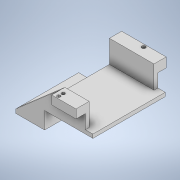
# Autodesk Inventor part: tray2
Saved by Autodesk Inventor 2020 (Build 240168000, 168)
## iProperties
Created: 2022-07-19
Part Number: tray2
Material: 일반
Document SubType Name: Modeling
Designer: SeungJin
Density: 1 g/cm^3
Appearance: 기본값
Author: SeungJin
Autodesk Inventor part; units mm, degrees
ref_plane "YZ Plane" through (0, 0, 0) normal (1, 0, 0) x (0, 1, 0)
ref_plane "XZ Plane" through (0, 0, 0) normal (0, 1, 0) x (-1, 0, 0)
ref_plane "XY Plane" through (0, 0, 0) normal (0, 0, 1) x (1, 0, 0)
sketch "스케치1" plane through (0, 0, 0) normal (0, 1, 0) x (-1, 0, 0)
  line L0 (70.5, 0) -> (70.5, 50)
  line L1 (70.5, 50) -> (0, 50)
  line L2 (0, 50) -> (0, 0)
  line L3 (24.5, 232.5) -> (-40, 232.5)
  line L4 (10, 242.5) -> (37.5, 242.5)
  line L5 (10, 232.5) -> (10, 242.5)
  line L6 (145.5, 232.5) -> (85.5, 232.5)
  line L7 (145.5, 242.5) -> (145.5, 232.5)
  line L8 (85.5, 242.5) -> (145.5, 242.5)
  line L9 (85.5, 232.5) -> (85.5, 242.5)
  line L10 (145.5, 0) -> (145.5, 242.5)
  line L11 (145.5, 242.5) -> (0, 242.5)
  line L12 (0, 242.5) -> (0, 0)
  line L13 (0, 50) -> (145.5, 50)
  circle A0 centre (93.5, 13) radius 2.067
  circle A1 centre (93.5, 37) radius 2.067
  circle A2 centre (147.5, 37) radius 2.067
  circle A3 centre (147.5, 13) radius 2.067
  line L14 (70.5, 0) -> (70.5, 50)
  line L15 (145.5, 50) -> (145.5, 81)
  line L16 (145.5, 75) -> (70.5, 75)
  line L17 (70.5, 50) -> (70.5, 75)
  line L18 (0, 0) -> (0, 25)
  line L19 (145.5, 27.5) -> (0, 27.5)
  line L20 (145.5, 0) -> (145.5, 25)
  line L21 (60.5, 242.5) -> (60.5, 267.5)
  line L22 (60.5, 267.5) -> (27.5, 267.5)
  line L23 (27.5, 267.5) -> (-42.5, 267.5)
  line L24 (145.5, 65) -> (-40, 65)
  circle A4 centre (12.5, 35) radius 2.067
  circle A5 centre (12.5, 15) radius 2.067
  circle A6 centre (-25, 256.5) radius 4.188
  circle A7 centre (12.5, 261) radius 2.067
  circle A8 centre (12.5, 249) radius 2.067
  line L25 (27.5, 242.5) -> (60.5, 242.5)
  line L26 (-40, 242.5) -> (20.5, 242.5)
  line L27 (0, 27.5) -> (0, 65)
  line L28 (145.5, 65) -> (145.5, 27.5)
  line L29 (0, 0) -> (145.5, 0)
  line L30 (24.5, 242.5) -> (24.5, 232.5)
  line L31 (0.5, 232.5) -> (0.5, 242.5)
  line L32 (113.5, 285) -> (113.5, 189)
  line L33 (39.5, 232.5) -> (39.5, 242.5)
  line L34 (39.5, 232.5) -> (24.5, 232.5)
  line L35 (-40, 242.5) -> (-40, 65)
  line L36 (-17.5, 242.5) -> (-17.5, 232.5)
  line L37 (0, 50) -> (-40, 50)
  line L38 (-40, 50) -> (-40, 65)
  line L39 (78.5, 75) -> (78.5, 0)
  point P0 (0, 227.5)
  point P1 (70.5, -15)
  point P2 (145.5, 227.5)
  point P3 (85.5, 242.5)
  point P4 (27.5, 242.5)
  point P5 (70.5, 25)
  point P6 (-5, 242.5)
  point P7 (0, 50)
  point P8 (70.5, 65)
  point P9 (0, 50)
  point P10 (78.5, 50)
  dimension "d1" = 50
  dimension "d3" = 4.134
  dimension "d4" = 4.134
  dimension "d5" = 4.134
  dimension "d6" = 4.134
  dimension "d7" = 12
  dimension "d8" = 12
  dimension "d9" = 32
  dimension "d10" = 15
  dimension "d29" = 40
  dimension "d30" = 30
  dimension "d97" = 10
  dimension "d98" = 10
  dimension "d101" = 8
  constraints: 78 end point, 11 point on line, 9 centre point, 8 vertical, 2 horizontal, 1 midpoint, 1 perpendicular, 14 other
  measures "d1" distance from line of L16 point (70.5, 25)
  measures "d3" diameter of A5
  measures "d4" diameter of A4
  measures "d5" diameter of A8
  measures "d6" diameter of A7
  measures "d7" distance from line of L30 A8.centre
  measures "d8" distance from line of A8.centre L31
  measures "d9" distance between parallel lines of L32 L10
  measures "d10" distance between parallel lines of L33 L30
  measures "d29" distance between parallel lines of L35 L12
  measures "d30" distance from line of L36 A8.centre
  measures "d98" distance between parallel lines of L8 L6
  measures "d101" distance between parallel lines of L39 L17
extrude "돌출1" add sketch "스케치1" against normal blind 10 contours L17 L24 L39 L13 | L1 L12 L24 L17 | L37 L38 L24 L12 | L24 L12 L3 L34 L33 L11 L9 L6 L10 L16 L17 | L17 L16 L39 L24 | L24 L35 L3 L12 | L12 L11 L31 L3 | L3 L36 L26 L12 | L31 L11 L5 L3 | L3 L35 L26 L36 | L5 L4 L30 L3 | L30 L4 L11 L33 L34 | L6 L32 L8 L7 | L6 L9 L8 L32
extrude "돌출2" add sketch "스케치1" along normal blind 82.3 contours L12 L11 L31 L3 | L3 L36 L26 L12 | L31 L11 L5 L3 | L3 L35 L26 L36 | L5 L4 L30 L3
sketch "스케치2" plane through (0, 82.3, 0) normal (0, 1, 0) x (1, 0, 0)
  line L0 (-24.5, -242.5) -> (40, -242.5) projected
  line L1 (40, -232.5) -> (-24.5, -232.5) projected
  line L2 (-24.5, -232.5) -> (40, -232.5) projected
  line L3 (-24.5, -242.5) -> (7.5, -242.5)
  line L4 (7.5, -232.5) -> (-24.5, -232.5)
  line L5 (-24.5, -232.5) -> (-24.5, -242.5)
  line L6 (40, -242.5) -> (40, -232.5) projected
  line L7 (7.5, -242.5) -> (7.5, -232.5)
  circle A0 centre (-12.5, -261) radius 2.067 projected
  circle A1 centre (-12.5, -249) radius 2.067 projected
  line L8 (-27.5, -267.5) -> (42.5, -267.5) projected
  circle A2 centre (25, -256.5) radius 4.188 projected
  line L9 (-24.5, -232.5) -> (40, -232.5)
  line L10 (40, -232.5) -> (40, -267.5)
  line L11 (40, -267.5) -> (-24.5, -267.5)
  line L12 (-24.5, -267.5) -> (-24.5, -232.5)
  line L13 (-24.5, -232.5) -> (-24.5, -242.5) projected
  point P0 (-0.5, -227.5)
  point P1 (0, -27.5)
  point P2 (7.5, -232.5)
  point P3 (40, -242.5)
  dimension "d31" = 20
  dimension "d48" = 12
  constraints: 16 end point, 3 parallel, 3 point on line, 2 horizontal, 1 perpendicular, 1 vertical, 3 other
  measures "d31" distance from line of L7 point (-12.5, -249)
  measures "d48" distance from line of L5 point (-12.5, -249)
extrude "돌출7" add sketch "스케치2" along normal blind 23 contours L5 L1 L7 L0 | L0 L10 L8 L12 | L7 L1 L6 L0 | A0 | A1 | A2
sketch "스케치16" plane through (0, 0, 0) normal (0, 1, 0) x (1, 0, 0)
  line L0 (-145.7919, -60) -> (40, -60)
  line L1 (-70.5, -50) -> (0, -50) projected
  line L2 (0, -50) -> (40, -50) projected
  line L3 (40, -50) -> (40, -60)
  line L4 (40, -50) -> (-80.5, -50) projected
  line L5 (-78.5, -50) -> (-78.5, -75) projected
  point P0 (0, 0)
  point P1 (-79.7, -60)
  point P2 (-78.5, -60)
  dimension "d96" = 10
  constraints: 4 end point, 1 other
  measures "d96" distance between parallel lines of L0 L2
extrude "돌출15" add sketch "스케치16" along normal blind 80
sketch "스케치10" plane through (40, 0, 232.5) normal (0, 0, -1) x (-1, 0, 0)
  line L0 (64.5, 82.3) -> (64.5, 105.3) projected
  line L1 (64.5, 0) -> (64.5, 82.3) projected
  line L2 (185.5, 0) -> (64.5, 0) projected
  line L3 (64.5, 105.3) -> (185.5, 0)
  point P0 (40, 0)
  constraints: 2 end point
extrude "돌출11" add sketch "스케치10" against normal up to surface (10 mm away)
sketch "스케치17" plane through (0, 80, 0) normal (0, 1, 0) x (1, 0, 0)
  line L0 (-145.5, -27.5) -> (0, -27.5) projected
  line L1 (0, -50) -> (0, 0) projected
  line L2 (-70.5, 0) -> (-70.5, -50) projected
  line L3 (-78.5, -60) -> (40, -60) projected
  circle A0 centre (-12.5, -35) radius 2.067 projected
  line L4 (40, -60) -> (-78.5, -60) projected
  line L5 (0, -60) -> (-90, -60)
  line L6 (-90, -60) -> (-90, -27.5)
  line L7 (-90, -27.5) -> (0, -27.5)
  line L8 (0, -27.5) -> (0, -60)
  line L9 (40, -232.5) -> (40, -60) projected
  line L10 (40, -60) -> (40, -27.5)
  line L11 (40, -27.5) -> (0, -27.5)
  line L12 (-78.5, -60) -> (-78.5, -27.5)
  point P0 (0, 0)
  point P1 (-70.5, -60)
  point P2 (0, -60)
  point P3 (0, -60)
  point P4 (0, -27.5)
  point P5 (-78.5, -27.5)
  dimension "d102" = 78.5
  constraints: 14 end point, 3 point on line, 2 parallel, 2 perpendicular, 2 vertical, 1 horizontal
  measures "d102" distance between parallel lines of L1 L12
extrude "돌출16" add sketch "스케치17" along normal blind 25.3 contours L0 L1 L8 L3 L12 | L11 L10 L3 L8 L1 | A0
sketch "스케치7" plane through (0, 105.3, 0) normal (0, 1, 0) x (1, 0, 0)
  point P0 (0, 0)
  point P1 (-12.5, -35)
hole "구멍1" at (-12.5, 105.3, 35) direction (0, -1, 0) diameter 5.5 end through all counterbore diameter 10 counterbore depth 15 clearance for "Hex Head Cap Screw ISO 24017" size "M5" standard "ISO"
sketch "스케치18" plane through (0, 105.3, 0) normal (0, 1, 0) x (1, 0, 0)
  line L0 (-12.5, -262) -> (-12.5, -260) construction
  line L1 (-7.5, -262) -> (-7.5, -260)
  line L2 (-17.5, -260) -> (-17.5, -262)
  arc A0 (-17.5, -262) -> (-7.5, -262) centre (-12.5, -262) ccw
  line L3 (-12.5, -262) -> (-12.5, -260) construction
  line L4 (-9.75, -262) -> (-9.75, -260)
  line L5 (-15.25, -260) -> (-15.25, -262)
  arc A1 (-15.25, -262) -> (-9.75, -262) centre (-12.5, -262) ccw
  arc A2 (-9.75, -260) -> (-15.25, -260) centre (-12.5, -260) ccw
  line L6 (-12.5, -250) -> (-12.5, -248) construction
  line L7 (-9.75, -250) -> (-9.75, -248)
  line L8 (-15.25, -248) -> (-15.25, -250)
  arc A3 (-15.25, -250) -> (-9.75, -250) centre (-12.5, -250) ccw
  arc A4 (-9.75, -248) -> (-15.25, -248) centre (-12.5, -248) ccw
  line L9 (-12.5, -250) -> (-12.5, -248) construction
  line L10 (-7.5, -250) -> (-7.5, -248)
  line L11 (-17.5, -248) -> (-17.5, -250)
  arc A5 (-7.5, -248) -> (-17.5, -248) centre (-12.5, -248) ccw
  line L12 (-17.5, -261) -> (-17.5, -249)
  line L13 (-7.5, -261) -> (-7.5, -249)
  circle A6 centre (-12.5, -261) radius 4
  line L14 (-16.5, -258.6906) -> (-12.5, -256.3812)
  line L15 (-12.5, -256.3812) -> (-8.5, -258.6906)
  line L16 (-8.5, -258.6906) -> (-8.5, -263.3094)
  line L17 (-8.5, -263.3094) -> (-12.5, -265.6188)
  line L18 (-12.5, -265.6188) -> (-16.5, -263.3094)
  line L19 (-16.5, -263.3094) -> (-16.5, -258.6906)
  circle A7 centre (-12.5, -249) radius 4
  line L20 (-16.5, -246.6906) -> (-12.5, -244.3812)
  line L21 (-12.5, -244.3812) -> (-8.5, -246.6906)
  line L22 (-8.5, -246.6906) -> (-8.5, -251.3094)
  line L23 (-8.5, -251.3094) -> (-12.5, -253.6188)
  line L24 (-12.5, -253.6188) -> (-16.5, -251.3094)
  line L25 (-16.5, -251.3094) -> (-16.5, -246.6906)
  point P0 (0, 0)
  point P1 (-16.5, -261)
  point P2 (-16.5, -249)
  dimension "d87" = 8
  dimension "d88" = 8
  constraints: 60 end point, 12 point on circle, 12 tangent, 6 centre point, 6 equal length, 6 midpoint, 4 coincident, 2 horizontal alignment, 1 point on line, 1 vertical, 30 other
extrude "돌출18" cut sketch "스케치18" against normal blind 15 contours A1 L5 A2 L4 | A3 L8 A4 L7 | A6 | L16 L17 A6 | A6 L15 L16 | A6 L14 L15 | L17 L18 A6 | A6 L19 L14 | L18 L19 A6 | A7 | L22 L23 A7 | A7 L21 L22 | A7 L20 L21 | L23 L24 A7 | A7 L25 L20 | L24 L25 A7
sketch "스케치20" plane through (0, 90.3, 0) normal (0, 1, 0) x (1, 0, 0)
  line L0 (-8.5, -258.6906) -> (-8.5, -263.3094) projected
  line L1 (-12.5, -256.3812) -> (-8.5, -258.6906) projected
  line L2 (-16.5, -258.6906) -> (-12.5, -256.3812) projected
  line L3 (-16.5, -263.3094) -> (-16.5, -258.6906) projected
  line L4 (-12.5, -265.6188) -> (-16.5, -263.3094) projected
  line L5 (-8.5, -263.3094) -> (-12.5, -265.6188) projected
  line L6 (-12.5, -244.3812) -> (-8.5, -246.6906) projected
  line L7 (-16.5, -246.6906) -> (-12.5, -244.3812) projected
  line L8 (-16.5, -251.3094) -> (-16.5, -246.6906) projected
  line L9 (-12.5, -253.6188) -> (-16.5, -251.3094) projected
  line L10 (-8.5, -251.3094) -> (-12.5, -253.6188) projected
  line L11 (-8.5, -246.6906) -> (-8.5, -251.3094) projected
  point P0 (0, 0)
  point P1 (-12.5, -261)
  point P2 (-12.5, -249)
hole "구멍3" at (-12.5, 90.3, 261) at (-12.5, 90.3, 249) direction (0, -1, 0) diameter 5.5 end through all clearance for "Hex Head Cap Screw ISO 24017" size "M5" standard "ISO"
sketch "스케치21" plane through (0, 0, 0) normal (0, 1, 0) x (1, 0, 0)
  line L0 (-145.5, -232.5) -> (40, -232.5) projected
  line L1 (40, -232.5) -> (40, -60) projected
  line L2 (40, -60) -> (-78.5, -60) projected
  line L3 (-78.5, -75) -> (-145.5, -75) projected
  line L4 (-145.5, -75) -> (-145.5, -232.5) projected
  line L5 (-145.5, -232.5) -> (-24.5, -232.5) projected
  line L6 (-145.5, -232.5) -> (-78.5, -232.5)
  line L7 (-78.5, -232.5) -> (-78.5, -81.5)
  line L8 (-78.5, -81.5) -> (-145.5, -81.5)
  line L9 (-145.5, -81.5) -> (-145.5, -232.5)
  line L10 (-78.5, -60) -> (-78.5, -75) projected
  line L11 (-68.5, -60) -> (-68.5, -232.5)
  line L12 (-78.5, -75) -> (-78.5, -50) projected
  line L13 (-78.5, -81.5) -> (-78.5, -60)
  line L14 (-78.5, -75) -> (-68.5, -75)
  point P0 (0, 0)
  point P1 (-68.5, -232.5)
  dimension "d99" = 67
  dimension "d100" = 151
  dimension "d103" = 10
  constraints: 14 end point, 4 perpendicular, 4 point on line, 2 parallel, 1 horizontal
  measures "d99" distance of L8.end L7.end
  measures "d100" distance of L7.end L6.end
  measures "d103" distance between parallel lines of L11 L7
extrude "돌출20" add sketch "스케치21" along normal blind 35 contours L7 L13 L14 L11 L0 | L14 L10 L2 L11
sketch "스케치23" plane through (0, 35, 0) normal (0, 1, 0) x (1, 0, 0)
  line L0 (-68.5, -232.5) -> (-68.5, -60) projected
  line L1 (-78.5, -60) -> (-68.5, -60) projected
  line L2 (-68.5, -232.5) -> (-78.5, -232.5) projected
  line L3 (-78.5, -60) -> (-78.5, -232.5) projected
  line L4 (40, -50) -> (40, -242.5) projected
  line L5 (-78.5, -60) -> (40, -60)
  line L6 (40, -60) -> (40, -232.5)
  line L7 (40, -232.5) -> (-78.5, -232.5)
  line L8 (-78.5, -232.5) -> (-78.5, -60)
  point P0 (0, 0)
  constraints: 8 end point, 2 parallel, 1 horizontal, 1 perpendicular, 1 point on line
extrude "돌출21" add sketch "스케치23" along normal blind 10
sketch "스케치25" plane through (40, 82.3, 267.5) normal (1, 0, 0) x (0, 0, -1)
  line L0 (217.5, -2.3) -> (217.5, -92.3) projected
  line L1 (217.5, -2.3) -> (240, -2.3) projected
  line L2 (207.5, 23) -> (240, 23) projected
  line L3 (207.5, -37.3) -> (207.5, 23) projected
  line L4 (35, -37.3) -> (35, 23) projected
  line L5 (0, 23) -> (35, 23) projected
  line L6 (0, 0) -> (0, 23) projected
  line L7 (0, 0) -> (25, 0) projected
  line L8 (25, -92.3) -> (25, 0) projected
  line L9 (35, -37.3) -> (35, -82.3) projected
  line L10 (35, -37.3) -> (25, -37.3)
  line L11 (207.5, -37.3) -> (217.5, -37.3)
  line L12 (217.5, -92.3) -> (25, -92.3) projected
  line L13 (35, -82.3) -> (207.5, -82.3) projected
  line L14 (240, -2.3) -> (240, 23) projected
  line L15 (207.5, -82.3) -> (207.5, -47.3) projected
  line L16 (35, -82.3) -> (35, -47.3) projected
  line L17 (35, -47.3) -> (207.5, -47.3) projected
  line L18 (35, -37.3) -> (207.5, -37.3) projected
  line L19 (35, -47.3) -> (25, -47.3)
  line L20 (25, -92.3) -> (25, 0) projected
  line L21 (207.5, -47.3) -> (217.5, -47.3)
  line L22 (217.5, -2.3) -> (217.5, -92.3) projected
  point P0 (267.5, -82.3)
  constraints: 8 end point, 4 point on line, 1 horizontal, 1 midpoint, 1 perpendicular
extrude "돌출23" add sketch "스케치25" along normal blind 20 contours L0 L21 L17 L9 L18 L11 | L9 L19 L8 L10
sketch "스케치27" plane through (0, -10, 0) normal (0, -1, 0) x (1, 0, 0)
  line L0 (-68.5, 232.5) -> (-68.5, 60) projected
  line L1 (40, 60) -> (-68.5, 60) projected
  line L2 (60, 242.5) -> (60, 50) projected
  line L3 (-68.5, 232.5) -> (40, 232.5) projected
  line L4 (40, 242.5) -> (-145.5, 242.5) projected
  line L5 (60, 242.5) -> (60, 232.5)
  line L6 (-78.5, 50) -> (40, 50) projected
  line L7 (60, 60) -> (60, 50)
  line L8 (-68.5, 232.5) -> (60, 232.5) projected
  line L9 (-68.5, 232.5) -> (-68.5, 242.5)
  line L10 (-68.5, 60) -> (-68.5, 50)
  line L11 (-78.5, 75) -> (-78.5, 50) projected
  line L12 (-145.5, 75) -> (-78.5, 75) projected
  line L13 (-78.5, 75) -> (-68.5, 75)
  line L14 (-68.5, 60) -> (-68.5, 232.5) projected
  line L15 (40, 50) -> (40, 60) projected
  line L16 (40, 50) -> (60, 50) projected
  line L17 (40, 242.5) -> (60, 242.5) projected
  line L18 (40, 232.5) -> (40, 242.5) projected
  point P0 (0, 0)
  point P1 (60, 232.5)
  point P2 (40, 232.5)
  point P3 (40, 232.5)
  constraints: 10 end point, 3 point on line, 3 vertical, 1 horizontal, 1 perpendicular
extrude "돌출24" cut sketch "스케치27" against normal up to surface (45 mm away) contours L3 L8 L2 L16 L15 L1 L0 | L9 L4 L18 L3 | L0 L10 L6 L11 L13 | L1 L15 L6 L10
